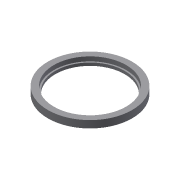
# Autodesk Inventor part: Cap
Saved by Autodesk Inventor 2015 (Build 190159000, 159)
## iProperties
Created: 2014-07-08
Part Number: Cap
Material: Generic
Document SubType Name: Modeling
Designer: I Rabey
Density: 1 g/cm^3
Appearance: Default
Author: I Rabey
Autodesk Inventor part; units mm, degrees
ref_plane "XY Plane" through (0, 0, 0) normal (0, 0, 1) x (1, 0, 0)
sketch "Sketch14" plane through (0, 0, 0) normal (0, 1, 0) x (-1, 0, 0)
  circle A0 centre (0, 0) radius 24
  circle A1 centre (0, 0) radius 29.1
  dimension "d122" = 48
  dimension "d123" = 58.2
  constraints: 2 centre point, 2 coincident
  measures "d122" diameter of A0
  measures "d123" diameter of A1
extrude "Extrusion3" add sketch "Sketch14" along normal blind 2
ref_plane "Work Plane1" through (0, 4.1, 0) normal (0, 1, 0) x (-1, 0, 0)
ref_plane "Work Plane2" through (29.5, 0, 0) normal (1, 0, 0) x (0, 1, 0)
ref_plane "Work Plane3" through (-29.5, 0, 0) normal (1, 0, 0) x (0, 1, 0)
sketch "Sketch22" plane through (0, 2, 0) normal (0, 1, 0) x (1, 0, 0)
  circle A0 centre (0, 0) radius 29.1
  circle A1 centre (0, 0) radius 25
  dimension "d188" = 58.2
  dimension "d189" = 50
  constraints: 2 centre point, 2 coincident
  measures "d188" diameter of A0
  measures "d189" diameter of A1
extrude "Extrusion7" add sketch "Sketch22" along normal blind 3
body "Solid3"
